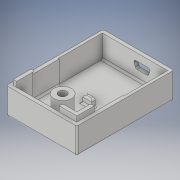
# Autodesk Inventor part: BoxLid2
Saved by Autodesk Inventor 2019 (Build 230136000, 136)
## iProperties
Created: 2020-09-23
Part Number: BoxLid2
Material: Generic
Document SubType Name: Modeling
Designer: Vincent
Density: 1 g/cm^3
Appearance: Default
Author: Vincent
Autodesk Inventor part; units mm, degrees
ref_plane "YZ Plane" through (0, 0, 0) normal (1, 0, 0) x (0, 1, 0)
ref_plane "XZ Plane" through (0, 0, 0) normal (0, 1, 0) x (-1, 0, 0)
ref_plane "XY Plane" through (0, 0, 0) normal (0, 0, 1) x (1, 0, 0)
sketch "Sketch1" plane through (0, 0, 0) normal (0, 1, 0) x (-1, 0, 0)
  line L0 (0, 0) -> (-40, 0)
  line L1 (-40, 0) -> (-40, -55)
  line L2 (-40, -55) -> (0, -55)
  line L3 (0, -55) -> (0, 0)
  dimension "d0" = 40
  dimension "d1" = 55
  constraints: 8 end point, 2 parallel, 1 horizontal, 1 perpendicular
  measures "d0" distance of L2.end L1.end
  measures "d1" distance of L1.end L0.end
extrude "Extrusion1" add sketch "Sketch1" along normal blind 15
shell "Shell1" thickness 2 removed faces 1 at (26.6667, 15, -18.3333)
sketch "Sketch2" plane through (2, 2, -2) normal (0, 1, 0) x (1, 0, 0)
  line L0 (36, 51) -> (36, 0) projected
  line L1 (36, 0) -> (26, 0)
  line L2 (26, 0) -> (26, 2)
  line L3 (26, 2) -> (36, 2)
  line L4 (36, 2) -> (36, 0)
  line L5 (36, 0) -> (34, 0)
  line L6 (34, 0) -> (34, 10)
  line L7 (34, 10) -> (36, 10)
  line L8 (36, 10) -> (36, 0)
  line L9 (0, 51) -> (0, 0) projected
  line L10 (0, 0) -> (2, 0)
  line L11 (2, 0) -> (2, 10)
  line L12 (2, 10) -> (0, 10)
  line L13 (0, 10) -> (0, 0)
  point P0 (-2, -2)
  dimension "d5" = 10
  dimension "d6" = 2
  dimension "d7" = 2
  dimension "d8" = 10
  dimension "d15" = 2
  dimension "d16" = 10
  constraints: 24 end point, 6 parallel, 3 horizontal, 3 perpendicular
  measures "d5" distance of L2.end L3.end
  measures "d6" distance of L1.end L2.end
  measures "d7" distance of L6.end L7.end
  measures "d8" distance of L5.end L6.end
  measures "d15" distance of L12.end L11.end
  measures "d16" distance of L11.end L10.end
extrude "Extrusion2" add sketch "Sketch2" along normal blind 16
sketch "Sketch3" plane through (2, 2, -53) normal (0, 1, 0) x (1, 0, 0)
  circle A0 centre (18, -41) radius 5
  line L0 (26, -51) -> (2, -51) projected
  line L1 (0, 0) -> (0, -41) projected
  line L2 (36, -41) -> (36, 0) projected
  point P0 (-2, -53)
  dimension "d17" = 10
  dimension "d18" = 10
  dimension "d19" = 18
  dimension "d20" = 18
  constraints: 1 centre point
  measures "d17" diameter of A0
  measures "d18" distance from line of L0 A0.centre
  measures "d19" distance from line of A0.centre L1
  measures "d20" distance from line of L2 A0.centre
extrude "Extrusion3" add sketch "Sketch3" along normal blind 13
sketch "Sketch4" plane through (0, 0, 0) normal (0, -1, 0) x (1, 0, 0)
  circle A0 centre (20, -12) radius 5 projected
  circle A1 centre (20, -12) radius 2.25
  circle A2 centre (20, -12) radius 4
  point P0 (0, 0)
  dimension "d23" = 4.5
  dimension "d24" = 8
  constraints: 2 centre point, 2 coincident
  measures "d23" diameter of A1
  measures "d24" diameter of A2
extrude "Extrusion4" cut sketch "Sketch4" against normal up to next contours A1
extrude "Extrusion5" cut sketch "Sketch4" against normal blind 8 contours A2
sketch "Sketch5" plane through (2, 2, -53) normal (0, 1, 0) x (1, 0, 0)
  line L0 (2, -51) -> (13, -51)
  line L1 (13, -51) -> (13, -45)
  line L2 (13, -45) -> (2, -45)
  line L3 (2, -45) -> (2, -51)
  line L4 (2, -51) -> (2, -41) projected
  line L5 (-2, 2) -> (-2, -53) projected
  line L6 (2, -51) -> (26, -51) projected
  dimension "d29" = 11
  dimension "d30" = 6
  dimension "d32" = 4
  constraints: 8 end point, 2 parallel, 1 horizontal, 1 perpendicular, 1 point on line
  measures "d29" distance of L2.end L1.end
  measures "d30" distance of L1.end L0.end
  measures "d32" distance between parallel lines of L5 L3
extrude "Extrusion6" cut sketch "Sketch5" against normal up to next
fillet "Fillet1" radius 1 9 edges at (20, 0, 0) (40, 0, -27.5) (0, 0, -27.5) (20, 0, -55) (16, 0, -12) (40, 7.5, -55) (0, 7.5, -55) (0, 7.5, 0) (40, 7.5, 0)
fillet "Fillet2" radius 2 1 edges at (15, 2, -12)
sketch "Sketch7" plane through (2, 2, -53) normal (0, 1, 0) x (1, 0, 0)
  line L0 (36.5, 0) -> (-0.5, 0)
  line L1 (-0.5, 0) -> (-0.5, -25)
  line L2 (-0.5, -25) -> (36.5, -25)
  line L3 (36.5, -25) -> (36.5, 0)
  line L4 (36, 0) -> (0, 0) projected
  line L5 (36, -41) -> (36, 0) projected
  line L6 (0, 0) -> (0, -41) projected
  line L7 (0, -41) -> (0, 0) projected
  line L8 (20.5, -25) -> (15.5, -25)
  line L9 (15.5, -25) -> (15.5, -27)
  line L10 (15.5, -27) -> (20.5, -27)
  line L11 (20.5, -27) -> (20.5, -25)
  point P0 (-2, -53)
  dimension "d39" = 25
  dimension "d40" = 0
  dimension "d42" = 0.5
  dimension "d43" = 0.5
  dimension "d46" = 5
  dimension "d47" = 2
  dimension "d48" = 15.5
  dimension "d49" = 15.5
  constraints: 16 end point, 4 parallel, 2 horizontal, 2 perpendicular, 1 point on line
  measures "d39" distance of L1.end L0.end
  measures "d40" distance between parallel lines of L4 L0
  measures "d42" distance between parallel lines of L5 L3
  measures "d43" distance between parallel lines of L7 L1
  measures "d46" distance of L10.end L9.end
  measures "d47" distance of L9.end L8.end
  measures "d48" distance between parallel lines of L5 L11
  measures "d49" distance between parallel lines of L6 L9
extrude "Extrusion7" cut sketch "Sketch7" along normal up to next contours L3 L2 L5 L0 | L5 L2 L6 L0 | L6 L2 L1 L0
extrude "Extrusion8" add sketch "Sketch7" along normal blind 4 contours L11 L10 L9 L2
fillet "Fillet3" radius 1 20 edges at (38, 8.5, -12) (36, 10, -12) (28, 8.5, -2) (28, 10, -4) (36, 10, -4) (2, 8.5, -12) (4, 10, -12) (32, 2, -4) (36, 2, -8) (4, 2, -10) (20, 2, -53) (38, 2, -20) (2, 2, -20) (21.5, 2, -2) (20, 2, -26) (17.5, 2, -27) (22.5, 2, -27) (17.5, 6, -27) (20, 6, -26) (22.5, 6, -27)
sketch "Sketch9" plane through (39, 15, -55) normal (0, 0, -1) x (-1, 0, 0)
  line L0 (20, -4) -> (10, -4)
  line L1 (10, -4) -> (11.5, -8)
  line L2 (11.5, -8) -> (18.5, -8)
  line L3 (18.5, -8) -> (20, -4)
  line L4 (0, -14) -> (0, 0) projected
  line L5 (38, 0) -> (38, -14) projected
  line L6 (38, -14) -> (0, -14) projected
  dimension "d54" = 10
  dimension "d55" = 4
  dimension "d58" = 10
  dimension "d63" = 7
  dimension "d66" = 1.5
  dimension "d70" = 6
  constraints: 8 end point, 1 parallel
  measures "d54" distance of L0.start L0.end
  measures "d55" distance between parallel lines of L0 L2
  measures "d58" distance from line of L4 L0.end
  measures "d63" distance of L1.end L2.end
  measures "d66" horizontal distance of L0.end L1.end
  measures "d70" distance between parallel lines of L6 L2
extrude "Extrusion9" cut sketch "Sketch9" against normal up to next
fillet "Fillet4" radius 1 4 edges at (20.5, 7, -54) (27.5, 7, -54) (19, 11, -54) (29, 11, -54)
equation "\"d19\" = d20"
equation "\"d48\" = d49"
body "Solid1"
